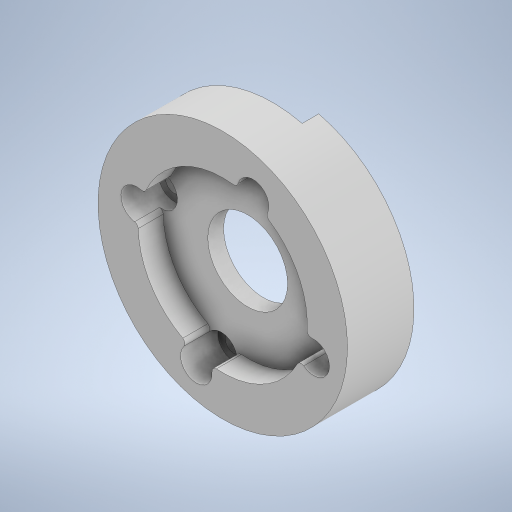
# Autodesk Inventor part: axis_4_top_frame
Saved by Autodesk Inventor 2024.1 (Build 281209000, 209)
## iProperties
Created: 2023-10-02
Part Number: axis_4_top_frame
Material: Generic
Document SubType Name: Modeling
Designer: chanh
Density: 1 g/cm^3
Appearance: Default
Author: chanh
Autodesk Inventor part; units mm, degrees
ref_plane "YZ Plane" through (0, 0, 0) normal (1, 0, 0) x (0, 1, 0)
ref_plane "XZ Plane" through (0, 0, 0) normal (0, 1, 0) x (-1, 0, 0)
ref_plane "XY Plane" through (0, 0, 0) normal (0, 0, 1) x (1, 0, 0)
sketch "Sketch1" plane through (0, 0, 0) normal (0, 0, 1) x (1, 0, 0)
  circle A0 centre (0, 0) radius 15
  dimension "d0" = 30
  constraints: 1 centre point, 1 coincident
  measures "d0" diameter of A0
extrude "Extrusion1" add sketch "Sketch1" along normal blind 8
sketch "Sketch2" plane through (0, 0, 0) normal (0, 0, -1) x (-1, 0, 0)
  circle A0 centre (0, 0) radius 6
  circle A1 centre (13.3002, 23.9784) radius 0.7835
  circle A2 centre (3.6379, 20.99) radius 0.7835
  circle A3 centre (15.8807, 14.1992) radius 0.7835
  circle A4 centre (-3.649, 9.9144) radius 0.7835
  circle A5 centre (10.3427, 2.1535) radius 0.7835
  line L0 (19.2874, 22.2584) -> (8.6711, 28.1469)
  line L1 (19.2874, 22.2584) -> (18.9381, 21.6287)
  arc A6 (18.9381, 21.6287) -> (19.717, 18.9097) centre (20.6871, 20.6586) ccw
  line L2 (19.717, 18.9097) -> (20.3466, 18.5604)
  line L3 (4.7764, -9.5105) -> (20.3466, 18.5604)
  line L4 (4.7764, -9.5105) -> (4.1468, -9.1613)
  arc A7 (4.1468, -9.1613) -> (1.4277, -9.9402) centre (3.1767, -10.9103) ccw
  line L5 (1.4277, -9.9402) -> (1.0784, -10.5698)
  line L6 (-9.5378, -4.6812) -> (1.0784, -10.5698)
  line L7 (-9.5378, -4.6812) -> (-9.1886, -4.0516)
  arc A8 (-9.1886, -4.0516) -> (-9.9674, -1.3325) centre (-10.9375, -3.0815) ccw
  line L8 (-9.9674, -1.3325) -> (-10.597, -0.9833)
  line L9 (4.9732, 27.0877) -> (-10.597, -0.9833)
  line L10 (4.9732, 27.0877) -> (5.6028, 26.7384)
  arc A9 (5.6028, 26.7384) -> (8.3219, 27.5173) centre (6.5729, 28.4874) ccw
  line L11 (8.3219, 27.5173) -> (8.6711, 28.1469)
  circle A10 centre (0, 0) radius 6.4
  arc A11 (3.081, -13.1443) -> (4.4406, -12.7549) centre (3.5661, -12.2698) ccw
  line L12 (0.4576, -11.6891) -> (3.081, -13.1443)
  line L13 (1.4277, -9.9402) -> (0.4576, -11.6891)
  arc A12 (4.1468, -9.1613) -> (1.4277, -9.9402) centre (3.1767, -10.9103) ccw
  line L14 (5.8957, -10.1314) -> (4.1468, -9.1613)
  line L15 (4.4406, -12.7549) -> (5.8957, -10.1314)
  circle A13 centre (3.1767, -10.9103) radius 0.7835
  circle A14 centre (-10.9375, -3.0815) radius 0.7835
  arc A15 (-13.1715, -2.9859) -> (-12.7821, -4.3454) centre (-12.2971, -3.4709) ccw
  line L16 (-11.7164, -0.3624) -> (-13.1715, -2.9859)
  line L17 (-9.9674, -1.3325) -> (-11.7164, -0.3624)
  arc A16 (-9.1886, -4.0516) -> (-9.9674, -1.3325) centre (-10.9375, -3.0815) ccw
  line L18 (-10.1587, -5.8006) -> (-9.1886, -4.0516)
  line L19 (-12.7821, -4.3454) -> (-10.1587, -5.8006)
  line L20 (21.466, 17.9395) -> (5.8957, -10.1314)
  line L21 (0.4576, -11.6891) -> (-10.1587, -5.8006)
  line L22 (-11.7164, -0.3624) -> (3.8539, 27.7085)
  arc A17 (4.0983, -9.2487) -> (1.5151, -9.9887) centre (3.1767, -10.9103) ccw
  line L23 (5.8472, -10.2188) -> (4.0983, -9.2487)
  line L24 (1.5151, -9.9887) -> (0.545, -11.7376)
  arc A18 (-9.276, -4.0031) -> (-10.0159, -1.42) centre (-10.9375, -3.0815) ccw
  line L25 (-10.0159, -1.42) -> (-11.7649, -0.4499)
  line L26 (-10.2461, -5.7521) -> (-9.276, -4.0031)
  line L27 (0.4965, -11.8251) -> (-10.2946, -5.8395)
  line L28 (21.5534, 17.891) -> (5.9347, -10.2674)
  line L29 (-11.8523, -0.4014) -> (3.7664, 27.757)
  line L30 (5.8472, -10.2188) -> (5.9347, -10.2674)
  line L31 (0.545, -11.7376) -> (0.4965, -11.8251)
  line L32 (-10.2461, -5.7521) -> (-10.2946, -5.8395)
  line L33 (-11.7649, -0.4499) -> (-11.8523, -0.4014)
  line L34 (4.9732, 27.0877) -> (3.7664, 27.757)
  line L35 (20.3466, 18.5604) -> (21.5534, 17.891)
  point P0 (0, 0)
extrude "Extrusion2" cut sketch "Sketch2" against normal blind 2 contours A0 | A4 | A5 | L1 A6 L2 L3 L4 A7 L5 L6 L7 A8 L8 L9 L10 A9 L11 L0 | L35 L20 L14 L3 | L9 L17 L22 L34 | L14 L15 L23 A17 L24 L12 L13 L5 A7 L4 | L35 L28 L30 L15 L20 | L8 A8 L7 L18 L19 L26 A18 L25 L16 L17 | L22 L16 L33 L29 L34 | L13 L21 L18 L6 | L12 L31 L27 L32 L19 L21 | A10
sketch "Sketch3" plane through (0, 0, 2) normal (0, 0, -1) x (-1, 0, 0)
  circle A0 centre (0, 0) radius 6.4 projected
  point P0 (0, 0)
extrude "Extrusion3" cut sketch "Sketch3" against normal blind 1.1
sketch "Sketch4" plane through (0, 0, 3.1) normal (0, 0, -1) x (-1, 0, 0)
  circle A0 centre (0, 0) radius 4.5 projected
  circle A1 centre (0, 0) radius 4.8
  dimension "d16" = 0.3
  constraints: 1 centre point
  measures "d16" radial gap between concentric circles of A0 A1
extrude "Extrusion4" cut sketch "Sketch4" against normal blind 10 contours A0 | A1
sketch "Sketch5" plane through (0, 0, 8) normal (0, 0, 1) x (1, 0, 0)
  circle A0 centre (0, 0) radius 9.96 projected
  circle A1 centre (0, 0) radius 10.16
  point P0 (0, 0)
  dimension "d19" = 0.2
  constraints: 1 centre point
  measures "d19" radial gap between concentric circles of A0 A1
extrude "Extrusion5" cut sketch "Sketch5" against normal blind 3 contours A0 | A1
sketch "Sketch6" plane through (0, 0, 8) normal (0, 0, 1) x (1, 0, 0)
  circle A0 centre (10.9375, -3.0815) radius 0.7835 projected
  circle A1 centre (-3.1767, -10.9103) radius 0.7835 projected
  circle A2 centre (-10.3427, 2.1535) radius 0.7835 projected
  circle A3 centre (3.649, 9.9144) radius 0.7835 projected
  point P0 (0, 0)
hole "Hole1" at (10.9375, -3.0815, 8) at (3.649, 9.9144, 8) at (-10.3427, 2.1535, 8) at (-3.1767, -10.9103, 8) direction (0, 0, -1) diameter 2.1 depth 8
sketch "Sketch7" plane through (0, 0, 8) normal (0, 0, 1) x (1, 0, 0)
  circle A0 centre (10.9375, -3.0815) radius 1.05 projected
  circle A1 centre (-3.1767, -10.9103) radius 1.05 projected
  arc A2 (-9.7097, 2.9912) -> (-10.0967, 1.1328) centre (-10.3427, 2.1535) ccw projected
  arc A3 (4.3847, 9.1652) -> (2.6032, 9.8208) centre (3.649, 9.9144) ccw projected
  circle A4 centre (10.9375, -3.0815) radius 1.9
  circle A5 centre (-3.1767, -10.9103) radius 1.9
  circle A6 centre (-10.3427, 2.1535) radius 1.9
  circle A7 centre (3.649, 9.9144) radius 1.9
  point P0 (0, 0)
  dimension "d29" = 3.8
  constraints: 4 centre point, 4 coincident, 3 equal radius
  measures "d29" diameter of A4
extrude "Extrusion6" cut sketch "Sketch7" against normal blind 4.5 contours A0 | A1 | A4 | A5 | A6 | A7
fillet "Fillet1" radius 0.5 8 edges at (9.3116, -4.0645, 6.5) (-1.4819, -10.0514, 6.5) (-4.1455, -9.2758, 6.5) (-10.1566, 0.2626, 6.5) (-9.4174, 3.8129, 6.5) (1.7513, 10.0079, 6.5) (5.1545, 8.7554, 6.5) (10.0639, -1.3943, 6.5)
body "Solid1"
